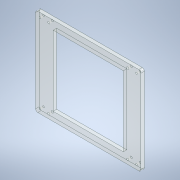
# Autodesk Inventor part: Heizelement_Grundplatte
Saved by Autodesk Inventor 2022 (Build 260153000, 153)
## iProperties
Created: 2021-12-03
Part Number: Heizelement_Grundplatte
Material: Glass
Document SubType Name: Modeling
Designer: domin
Density: 2.18 g/cm^3
Appearance: Clear
Mass: 471.747 g
Surface Area: 696.556 cm^2
Volume: 216.398 cm^3
Author: domin
Autodesk Inventor part; units mm, degrees
ref_plane "YZ Plane" through (0, 0, 0) normal (1, 0, 0) x (0, 1, 0)
ref_plane "XZ Plane" through (0, 0, 0) normal (0, 1, 0) x (-1, 0, 0)
ref_plane "XY Plane" through (0, 0, 0) normal (0, 0, 1) x (1, 0, 0)
sketch "Sketch1" plane through (0, 0, 0) normal (0, 0, 1) x (1, 0, 0)
  line L0 (-120, 100) -> (120, 100)
  line L1 (120, 100) -> (120, -100)
  line L2 (120, -100) -> (-120, -100)
  line L3 (-120, -100) -> (-120, 100)
  line L4 (-80, 80) -> (80, 80)
  line L5 (80, 80) -> (80, -80)
  line L6 (80, -80) -> (-80, -80)
  line L7 (-80, -80) -> (-80, 80)
  point P0 (0, 0)
  dimension "d0" = 240
  dimension "d1" = 200
  dimension "d2" = 120
  dimension "d3" = 100
  dimension "d4" = 160
  dimension "d5" = 160
  dimension "d6" = 80
  dimension "d7" = 80
  constraints: 16 end point, 4 parallel, 2 horizontal, 2 perpendicular
  measures "d0" distance between parallel lines of L1 L3
  measures "d1" distance between parallel lines of L2 L0
  measures "d2" distance from line of point (0, 0) L3
  measures "d3" distance from line of point (0, 0) L0
  measures "d4" distance between parallel lines of L5 L7
  measures "d5" distance between parallel lines of L6 L4
  measures "d6" distance from line of point (0, 0) L4
  measures "d7" distance from line of point (0, 0) L7
extrude "Extrusion1" add sketch "Sketch1" along normal mid plane 8
fillet "Fillet1" radius 5 4 edges at (-120, 100, 0) (-120, -100, 0) (120, -100, 0) (120, 100, 0)
sketch "Sketch2" plane through (0, 0, 4) normal (0, 0, 1) x (1, 0, 0)
  line L0 (-90, 90) -> (90, 90)
  line L1 (90, 90) -> (90, -90)
  line L2 (90, -90) -> (-90, -90)
  line L3 (-90, -90) -> (-90, 90)
  circle A0 centre (-90, 90) radius 2.5
  circle A1 centre (90, 90) radius 2.5
  circle A2 centre (90, -90) radius 2.5
  circle A3 centre (-90, -90) radius 2.5
  point P0 (0, 0)
  dimension "d11" = 180
  dimension "d12" = 180
  dimension "d13" = 90
  dimension "d14" = 90
  dimension "d15" = 5
  constraints: 8 end point, 4 centre point, 4 coincident, 3 equal radius, 2 parallel, 1 horizontal, 1 perpendicular
  measures "d11" distance between parallel lines of L1 L3
  measures "d12" distance between parallel lines of L2 L0
  measures "d13" distance from line of point (0, 0) L0
  measures "d14" distance from line of point (0, 0) L3
  measures "d15" diameter of A0
hole "Hole1" at (-90, 90, 4) at (90, 90, 4) at (90, -90, 4) at (-90, -90, 4) direction (0, 0, -1) diameter 5 end through all
sketch "Sketch3" plane through (0, 0, 4) normal (0, 0, 1) x (1, 0, 0)
  line L0 (-110, 90) -> (110, 90)
  line L1 (110, 90) -> (110, -90)
  line L2 (110, -90) -> (-110, -90)
  line L3 (-110, -90) -> (-110, 90)
  circle A0 centre (-110, 90) radius 2
  circle A1 centre (110, 90) radius 2
  circle A2 centre (110, -90) radius 2
  circle A3 centre (-110, -90) radius 2
  point P0 (0, 0)
  dimension "d23" = 220
  dimension "d24" = 180
  dimension "d25" = 110
  dimension "d26" = 90
  dimension "d27" = 4
  constraints: 8 end point, 4 centre point, 4 coincident, 3 equal radius, 2 parallel, 1 horizontal, 1 perpendicular
  measures "d23" distance between parallel lines of L1 L3
  measures "d24" distance between parallel lines of L2 L0
  measures "d25" distance from line of point (0, 0) L3
  measures "d26" distance from line of point (0, 0) L0
  measures "d27" diameter of A0
hole "Hole2" at (-110, 90, 4) at (110, 90, 4) at (110, -90, 4) at (-110, -90, 4) direction (0, 0, -1) diameter 4 end through all
equation "\"d2\" = 0.5 * d0"
equation "\"d3\" = 0.5 * d1"
equation "\"d6\" = 0.5 * d4"
equation "\"d7\" = 0.5 * d5"
equation "\"d12\" = d11"
equation "\"d13\" = 0.5 * d11"
equation "\"d14\" = 0.5 * d11"
equation "\"d16\" = d15"
equation "\"d25\" = 0.5 * d23"
equation "\"d26\" = 0.5 * d24"
equation "\"d28\" = d27"
body "Solid1"
